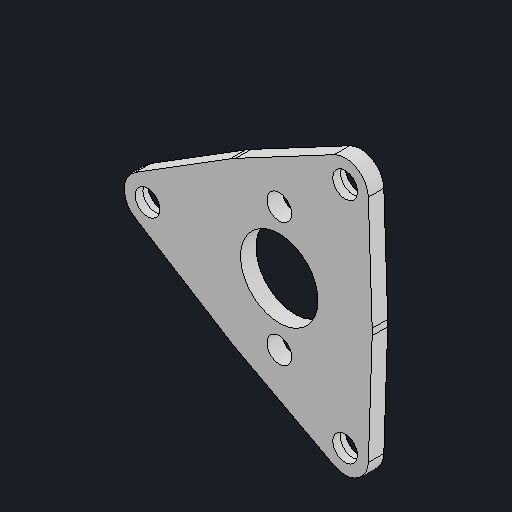
# Autodesk Inventor part: BLDC_mount
Saved by Autodesk Inventor 2024.2 (Build 282272000, 272)
## iProperties
Created: 2024-03-07
Part Number: BLDC_mount
Material: 一般
Document SubType Name: Modeling
Designer: Hanaoka
Density: 1 g/cm^3
Appearance: 既定
Author: Hanaoka
Autodesk Inventor part; units mm, degrees
ref_plane "YZ Plane" through (0, 0, 0) normal (1, 0, 0) x (0, 1, 0)
ref_plane "XZ Plane" through (0, 0, 0) normal (0, 1, 0) x (-1, 0, 0)
ref_plane "XY Plane" through (0, 0, 0) normal (0, 0, 1) x (1, 0, 0)
sketch "スケッチ1" plane through (0, 0, 0) normal (0, 0, 1) x (1, 0, 0)
  circle A0 centre (0, 0) radius 1.5 construction
  circle A1 centre (0, 8) radius 1.6
  circle A2 centre (0, 0) radius 8 construction
  circle A3 centre (0, -8) radius 1.6
  circle A4 centre (0, 0) radius 5
  circle A5 centre (0, 0) radius 14 construction
  circle A6 centre (-17, 0) radius 3
  circle A7 centre (8.5, 14.7224) radius 3
  circle A8 centre (8.5, -14.7224) radius 3
  circle A9 centre (0, 0) radius 12
  line L0 (11.4982, -14.8253) -> (11.9929, -0.4116)
  line L1 (11.9929, 0.4116) -> (11.4982, 14.8253)
  line L2 (-69.266, 0) -> (45.3789, 0) construction
  line L3 (34.633, -59.9861) -> (-22.6894, 39.2993) construction
  line L4 (34.633, 59.9861) -> (-22.6894, -39.2993) construction
  line L5 (7.09, 17.3704) -> (-5.64, 10.592)
  line L6 (-6.3529, 10.1804) -> (-18.5882, 2.5451)
  line L7 (-18.5882, -2.5451) -> (-6.3529, -10.1804)
  line L8 (7.09, -17.3704) -> (-5.64, -10.592)
  line L9 (-92.195, 0) -> (68.3079, 0) projected
  point P0 (5.868, 16.1622)
  point P1 (11.4335, -15.3506)
  point P2 (-14.8215, -2.0626)
  point P3 (-16.5273, -2.9625)
  point P4 (8.5, -14.7224)
  point P5 (8.5, 14.7224)
  point P6 (6.25, 10.8253)
  point P7 (6.25, -10.8253)
  dimension "d6" = 16
  dimension "d0" = 3
  dimension "d1" = 3.2
  dimension "d4" = 360
  dimension "d7" = 10
  dimension "d8" = 28
  dimension "d11" = 24
  dimension "d12" = 6
  dimension "d15" = 360
  constraints: 18 end point, 16 point on circle, 15 tangent, 9 centre point, 8 point on line, 5 coincident, 2 vertical alignment, 1 equal radius, 1 symmetric about line, 23 other
  measures "d0" diameter of A0
  measures "d1" diameter of A1
  measures "d7" diameter of A4
  measures "d8" diameter of A5
  measures "d11" diameter of A9
  measures "d12" diameter of A7
extrude "押し出し1" add sketch "スケッチ1" along normal blind 2 contours L9 A9 A4 | A4 L9 A9 | L9 A6 L6 A9 | A9 L7 A6 L9 | A9 L5 A7 L1 | L0 A8 L8 A9 | L9 A6 | A6 L9 | A7 | A8
hole "穴1" at (8.5, 14.7224, 0) at (-17, 0, 0) at (8.5, -14.7224, 0) direction (0, 0, 1) diameter 3.2 end through all counterbore diameter 4 counterbore depth 1
